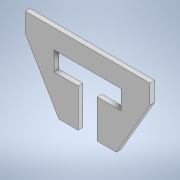
# Autodesk Inventor part: Assignment 3.1 - Latch Clip
Saved by Autodesk Inventor 2022 (Build 260153000, 153)
## iProperties
Created: 2021-05-23
Part Number: Assignment 3.1 - Latch Clip
Material: Generic
Document SubType Name: Modeling
Designer: Aaron
Density: 1 g/cm^3
Appearance: Default
Author: Aaron
Autodesk Inventor part; units mm, degrees
ref_plane "YZ Plane" through (0, 0, 0) normal (1, 0, 0) x (0, 1, 0)
ref_plane "XZ Plane" through (0, 0, 0) normal (0, 1, 0) x (-1, 0, 0)
ref_plane "XY Plane" through (0, 0, 0) normal (0, 0, 1) x (1, 0, 0)
sketch "Sketch1" plane through (0, 0, 0) normal (0, 0, 1) x (1, 0, 0)
  line L0 (0, 0) -> (25.4, 0)
  line L1 (25.4, 0) -> (25.4, 50.8)
  line L2 (25.4, 50.8) -> (-6.35, 50.8)
  line L3 (-6.35, 50.8) -> (-6.35, 76.2)
  line L4 (-6.35, 76.2) -> (82.55, 76.2)
  line L5 (82.55, 76.2) -> (82.55, 50.8)
  line L6 (82.55, 50.8) -> (50.8, 50.8)
  line L7 (50.8, 50.8) -> (50.8, 0)
  line L8 (50.8, 0) -> (76.2, 0)
  line L9 (120.65, 76.2) -> (76.2, 0)
  line L10 (120.65, 76.2) -> (120.65, 101.6)
  line L11 (120.65, 101.6) -> (-44.45, 101.6)
  line L12 (-44.45, 101.6) -> (-44.45, 76.2)
  line L13 (-44.45, 76.2) -> (0, 0)
  dimension "d0" = 25.4
  dimension "d1" = 50.8
  dimension "d2" = 31.75
  dimension "d3" = 25.4
  dimension "d4" = 88.9
  dimension "d5" = 25.4
  dimension "d6" = 31.75
  dimension "d7" = 25.4
  dimension "d10" = 25.4
  dimension "d11" = 165.1
  dimension "d12" = 25.4
  constraints: 28 end point, 7 perpendicular, 5 point on line, 1 horizontal, 1 vertical
  measures "d0" distance of L0.start L0.end
  measures "d1" distance of L0.end L1.end
  measures "d2" distance of L1.end L2.end
  measures "d3" distance of L2.end L3.end
  measures "d4" distance of L3.end L4.end
  measures "d5" distance of L4.end L5.end
  measures "d6" distance of L5.end L6.end
  measures "d7" distance of L7.end L8.end
  measures "d10" distance of L9.start L10.end
  measures "d11" distance of L10.end L11.end
  measures "d12" distance of L11.end L12.end
extrude "Extrusion1" add sketch "Sketch1" along normal blind 6.35
body "Solid1"
